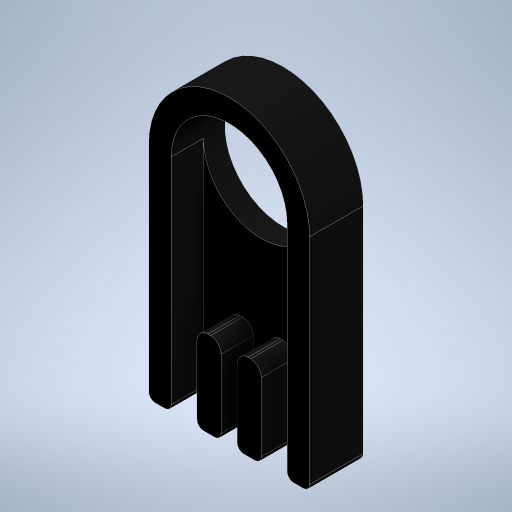
# Autodesk Inventor part: potentiometr_case
Saved by Autodesk Inventor 2024.2 (Build 282272000, 272)
## iProperties
Created: 2023-12-27
Part Number: potentiometr_case
Material: PLA
Document SubType Name: Modeling
Designer: Konrad
Density: 1 g/cm^3
Appearance: PLA
Author: Konrad
Autodesk Inventor part; units mm, degrees
ref_plane "YZ Plane" through (0, 0, 0) normal (1, 0, 0) x (0, 1, 0)
ref_plane "XZ Plane" through (0, 0, 0) normal (0, 1, 0) x (-1, 0, 0)
ref_plane "XY Plane" through (0, 0, 0) normal (0, 0, 1) x (1, 0, 0)
sketch "Szkic1" plane through (0, 0, 0) normal (0, 0, 1) x (1, 0, 0)
  circle A0 centre (0, 0) radius 5.4
  line L0 (0, 5.4) -> (0, -12.6) construction
  line L1 (-5.4, 0) -> (-5.4, -12.6)
  line L2 (1.75, -12.6) -> (5.4, -12.6) construction
  line L3 (5.4, -12.6) -> (5.4, 0)
  line L4 (-4.5, -12.6) -> (-4.5, -16.6)
  line L5 (-4.5, -16.6) -> (-3, -16.6)
  line L6 (-3, -16.6) -> (-3, -13.6)
  line L7 (-3, -12.6) -> (-4.5, -12.6)
  line L8 (-4.5, -12.6) -> (-3, -16.6) construction
  line L9 (-4.5, -16.6) -> (-3, -12.6) construction
  line L10 (0.75, -12.6) -> (-0.75, -12.6)
  line L11 (0.75, -16.6) -> (0.75, -13.6)
  line L12 (-0.75, -16.6) -> (0.75, -16.6)
  line L13 (-0.75, -12.6) -> (0.75, -16.6) construction
  line L14 (-0.75, -16.6) -> (0.75, -12.6) construction
  line L15 (-0.75, -13.6) -> (-0.75, -16.6)
  line L16 (4.5, -12.6) -> (3, -12.6)
  line L17 (4.5, -16.6) -> (4.5, -12.6)
  line L18 (3, -16.6) -> (4.5, -16.6)
  line L19 (3, -12.6) -> (4.5, -16.6) construction
  line L20 (3, -16.6) -> (4.5, -12.6) construction
  line L21 (3, -13.6) -> (3, -16.6)
  line L22 (-7.5, 7.5) -> (7.5, 7.5)
  line L23 (7.5, 7.5) -> (7.5, -20.6)
  line L24 (7.5, -20.6) -> (-7.5, -20.6)
  line L25 (-7.5, -20.6) -> (-7.5, 7.5)
  line L26 (5.4, 0) -> (5.4, -20.6)
  line L27 (5.4, -20.6) -> (-5.4, -20.6) construction
  line L28 (-5.4, -20.6) -> (-5.4, 0)
  line L29 (-3, -16.6) -> (-3, -20.6)
  line L30 (-0.75, -16.6) -> (-0.75, -20.6)
  line L31 (0.75, -16.6) -> (0.75, -20.6)
  line L32 (3, -16.6) -> (3, -20.6)
  line L33 (4.5, -16.6) -> (4.5, -20.6) construction
  line L34 (2, -12.6) -> (0.75, -12.6) construction
  line L35 (-3, -12.6) -> (-1.75, -12.6) construction
  arc A1 (-2, -12.6) -> (-3, -13.6) centre (-2, -13.6) ccw
  arc A2 (-0.75, -13.6) -> (-1.75, -12.6) centre (-1.75, -13.6) ccw
  arc A3 (1.75, -12.6) -> (0.75, -13.6) centre (1.75, -13.6) ccw
  arc A4 (3, -13.6) -> (2, -12.6) centre (2, -13.6) ccw
  line L36 (-2, -12.6) -> (-1.75, -12.6)
  line L37 (1.75, -12.6) -> (2, -12.6)
  line L38 (3, -13.6) -> (3, -16.6)
  line L39 (5.4, -16.6) -> (3, -16.6) construction
  line L40 (-3, -16.6) -> (-5.4, -16.6) construction
  line L41 (-3, -16.6) -> (-3, -13.6)
  line L42 (-0.75, -13.6) -> (-0.75, -16.6)
  line L43 (0.75, -16.6) -> (0.75, -13.6)
  circle A5 centre (0, 0) radius 7.5
  line L44 (-7.5, -7.5) -> (7.5, -7.5)
  point P0 (-3.75, -14.6)
  point P1 (0, -14.6)
  point P2 (3.75, -14.6)
  point P3 (0, -14.6)
  point P4 (0, -14.6)
  point P5 (0, 5.4)
  point P6 (-3, -20.5)
  point P7 (-0.75, -20.6)
  point P8 (0.75, -13.6)
  point P9 (0.75, -20.6)
  point P10 (3, -20.6)
  point P11 (5.4, -12.6)
  point P12 (0, 7.5)
  point P13 (7.5, 0)
  point P14 (-7.5, 0)
  point P15 (-5.4, -5.2048)
  point P16 (5.4, -5.2048)
  dimension "d29" = 15
  dimension "d0" = 10.8
  dimension "d3" = 12.6
  dimension "d5" = 4
  dimension "d6" = 1.5
  dimension "d9" = 3.75
  dimension "d16" = 1
  dimension "d28" = 15
  dimension "d30" = 28.1
  constraints: 91 end point, 25 point on line, 11 perpendicular, 11 point on circle, 10 tangent, 9 midpoint, 7 collinear, 5 centre point, 5 parallel, 3 coincident, 3 equal radius, 3 horizontal, 3 vertical, 26 other
  measures "d0" diameter of A0
  measures "d3" distance of L1.start L1.end
  measures "d5" distance of L4.start L4.end
  measures "d6" distance of L5.end L4.end
  measures "d9" distance of L4.start L10.end
  measures "d16" radius of A1
  measures "d28" distance of L22.end L22.start
  measures "d30" distance of L23.end L22.end
extrude "Wyciągnięcie proste1" add sketch "Szkic1" against normal blind 2 contours L3 A5 L1 A0 | A0 L1 A5 L3 | A5 L23 L44 L3 | L3 L44 A5 | A5 L44 L1 | L1 L44 L25 A5 | L44 L23 L24 L26 L3 | L3 L26 L24 L32 L21 A4 L37 A3 L11 L12 L15 A2 L36 A1 L6 L29 L28 L1 L44 | L1 L28 L24 L25 L44 | L24 L31 L11 A3 L37 A4 L21 L32 | L29 L6 A1 L36 A2 L15 L30 L24 | L24 L30 L12 L31
extrude "Wyciągnięcie proste2" add sketch "Szkic1" along normal blind 3 contours A0 L1 A5 L3 | A5 L23 L44 L3 | L1 L44 L25 A5 | L44 L23 L24 L26 L3 | L1 L28 L24 L25 L44 | L24 L31 L11 A3 L37 A4 L21 L32 | L29 L6 A1 L36 A2 L15 L30 L24 picked at (-5.6976, -3.095)
fillet "Zaokrąglenie1" radius 0.6 8 edges at (-7.5, -20.6, 0.5) (7.5, -20.6, 0.5) (-5.4, -20.6, 1.5) (5.4, -20.6, 1.5) (3, -20.6, 1.5) (0.75, -20.6, 1.5) (-3, -20.6, 1.5) (-0.75, -20.6, 1.5)
